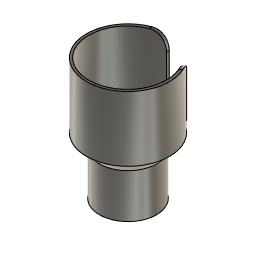
cupAdapter v1 (Autodesk Fusion 360 design; units mm, degrees)
Autodesk Fusion 360 part; units mm, degrees
note: some values were not read from the file. Set by a fixed rule: which sketch regions a step uses.
cylinder "CylinderPrimitive1" add diameter 69.85 height 69.85 placed x (1, 0, 0) y (0, 1, 0) z (0, 0, 1) at (0, 0, 0)
cylinder "CylinderPrimitive2" add diameter 101.6 height 79.375 placed x (1, 0, 0) y (0, 1, 0) z (0, 0, 1) at (0, 0, 69.85)
hole "Hole1" at (-0.2397, -0.2457, 149.225) direction (0, 0, -1) diameter 95.25 depth 76.2 tip angle 180
chamfer "Chamfer1" distance 15.875 angle 45 1 edges at (-32.5615, -12.6294, 69.85)
sketch "Sketch8" plane through (0, 0, 149.225) normal (0, 0, 1) x (-1, 0, 0)
  circle A0 centre (0.2397, 0.2457) radius 47.625
  circle A1 centre (0, 0) radius 50.8
  line L0 (0.2397, 0.2457) -> (0.2397, -50.7994)
  line L1 (0, 0) -> (-58.42, -58.42)
  constraint coincident A0.centre L0.start
  constraint coincident A1 L0.end
  constraint vertical L0
  constraint coincident A1.centre L1.start
extrude "Extrude1" cut sketch "Sketch8" against normal blind 76.2 contours A0 A1 L0 L1 picked at (-33.4159, -36.5603)
fillet "Fillet1" radius 17.78 4 edges at (34.6771, 34.6771, 73.025) (34.6771, 34.6771, 149.225) (-0.2397, 49.0894, 149.225) (-0.2397, 49.0894, 73.025)
